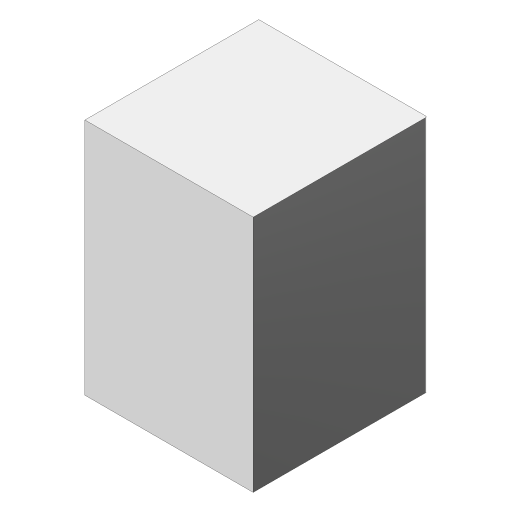
# Autodesk Inventor part: fridge
Saved by Autodesk Inventor 2023 (Build 270158000, 158)
## iProperties
Created: 2022-09-12
Part Number: fridge
Material: 常规
Document SubType Name: Modeling
Designer: byfbi
Density: 1 g/cm^3
Appearance: 默认
Author: byfbi
Autodesk Inventor part; units mm, degrees
ref_plane "YZ Plane" through (0, 0, 0) normal (1, 0, 0) x (0, 1, 0)
ref_plane "XZ Plane" through (0, 0, 0) normal (0, 1, 0) x (-1, 0, 0)
ref_plane "XY Plane" through (0, 0, 0) normal (0, 0, 1) x (1, 0, 0)
sketch "草图1" plane through (0, 0, 0) normal (1, 0, 0) x (0, 1, 0)
  line L0 (425, -310) -> (-425, -310)
  line L1 (-425, -310) -> (-425, 310)
  line L2 (-425, 310) -> (425, 310)
  line L3 (425, 310) -> (425, -310)
  line L4 (425, -310) -> (-425, 310) construction
  line L5 (-425, -310) -> (425, 310) construction
  point P0 (0, 0)
  dimension "d0" = 850
  dimension "d1" = 620
  constraints: 12 end point, 2 midpoint, 2 parallel, 1 horizontal, 1 perpendicular
  measures "d0" distance of L1.end L2.end
  measures "d1" distance of L0.end L1.end
extrude "拉伸1" add sketch "草图1" along normal blind 600
fillet "圆角1" radius 5 1 edges at (600, 0, -310)
